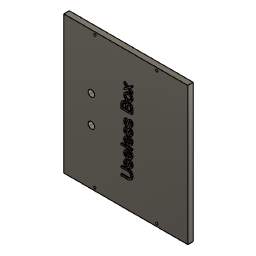
UselessBoxTop v6 (Autodesk Fusion 360 design; units mm, degrees)
Autodesk Fusion 360 part; units mm, degrees
note: some values were not read from the file. Set by a fixed rule: which sketch regions a step uses.
sketch "Sketch1" plane through (0, 0, 0) normal (0, 0, 1) x (1, 0, 0)
  line L0 (0, 0) -> (114.3, 0)
  line L1 (114.3, 0) -> (114.3, 127)
  line L2 (114.3, 127) -> (0, 127)
  line L3 (0, 127) -> (0, 0)
  dimension "d1" = 114.3
  dimension "d2" = 127
  constraint horizontal L0
  constraint vertical L1
  constraint horizontal L2
  constraint vertical L3
  constraint coincident L0.start L3.end
  measures "d1" distance of L0.start L0.end
  measures "d2" distance of L0.start L2.end
extrude "Extrude1" add sketch "Sketch1" along normal blind 5
sketch "Sketch2" plane through (0, 0, 5) normal (0, 0, 1) x (1, 0, 0)
  line L0 (0, 127) -> (0, 0)
  line L1 (0, 0) -> (114.3, 0)
  line L2 (114.3, 0) -> (114.3, 127)
  line L3 (114.3, 127) -> (0, 127)
  line L4 (0, 0) -> (114.3, 0)
  line L5 (114.3, 0) -> (114.3, 2.5)
  line L6 (114.3, 2.5) -> (0, 2.5)
  line L7 (0, 2.5) -> (0, 0)
  line L8 (0, 127) -> (114.3, 127)
  line L9 (114.3, 127) -> (114.3, 124.5)
  line L10 (114.3, 124.5) -> (0, 124.5)
  line L11 (0, 124.5) -> (0, 127)
  line L12 (0, 2.5) -> (28.575, 2.5)
  line L13 (28.575, 2.5) -> (28.575, 0)
  line L14 (28.575, 0) -> (0, 0)
  line L15 (0, 0) -> (0, 2.5)
  line L16 (114.3, 2.5) -> (85.725, 2.5)
  line L17 (85.725, 2.5) -> (85.725, 0)
  line L18 (85.725, 0) -> (114.3, 0)
  line L19 (114.3, 0) -> (114.3, 2.5)
  line L20 (0, 127) -> (28.575, 127)
  line L21 (28.575, 127) -> (28.575, 124.5)
  line L22 (28.575, 124.5) -> (0, 124.5)
  line L23 (0, 124.5) -> (0, 127)
  line L24 (114.3, 124.5) -> (85.725, 124.5)
  line L25 (85.725, 124.5) -> (85.725, 127)
  line L26 (85.725, 127) -> (114.3, 127)
  line L27 (114.3, 127) -> (114.3, 124.5)
  circle A0 centre (28.575, 124.5) radius 1.05
  circle A1 centre (85.725, 124.5) radius 1.05
  circle A2 centre (85.725, 2.5) radius 1.05
  circle A3 centre (28.575, 2.5) radius 1.05
  dimension "d5" = 114.3
  dimension "d6" = 2.5
  dimension "d7" = 114.3
  dimension "d8" = 2.5
  dimension "d9" = 28.575
  dimension "d10" = 28.575
  dimension "d11" = 28.575
  dimension "d12" = 28.575
  dimension "d13" = 2.1
  dimension "d14" = 2.1
  dimension "d15" = 2.1
  dimension "d16" = 2.1
  constraint horizontal L4
  constraint vertical L5
  constraint horizontal L6
  constraint vertical L7
  constraint coincident L0.end L1.start
  constraint horizontal L8
  constraint vertical L9
  constraint horizontal L10
  constraint vertical L11
  constraint coincident L0.start L3.end
  constraint horizontal L12
  constraint vertical L13
  constraint horizontal L14
  constraint vertical L15
  constraint horizontal L16
  constraint vertical L17
  constraint horizontal L18
  constraint vertical L19
  constraint horizontal L20
  constraint vertical L21
  constraint horizontal L22
  constraint vertical L23
  constraint horizontal L24
  constraint vertical L25
  constraint horizontal L26
  constraint vertical L27
  constraint coincident L21.end L22.start
  constraint coincident L24.end L25.start
  constraint coincident L16.end L17.start
  constraint coincident L12.end L13.start
  measures "d5" distance of L0.end L1.end
  measures "d6" distance of L0.end L6.end
  measures "d7" distance of L0.start L2.end
  measures "d8" distance of L0.start L10.end
  measures "d9" distance of L6.end L12.end
  measures "d10" distance of L5.end L16.end
  measures "d11" distance of L0.start L20.end
  measures "d12" distance of L9.end L24.end
  measures "d13" diameter of A0
  measures "d14" diameter of A1
  measures "d15" diameter of A2
  measures "d16" diameter of A3
extrude "Extrude2" cut sketch "Sketch2" against normal blind 5 contours L10 L21 L22 A0 | L10 L22 A0 | L10 L21 A0 | L6 L12 A3 | L6 L12 L13 A3 | L10 L24 L25 A1 | L10 L25 A1 | L6 L13 A3 | L10 L24 A1 | L6 L16 A2 | L6 L17 A2 | L6 L16 L17 A2
sketch "Sketch3" plane through (0, 0, 5) normal (0, 0, 1) x (1, 0, 0)
  circle A0 centre (85.725, 124.5) radius 1.05
  circle A1 centre (85.725, 2.5) radius 1.05
  circle A2 centre (28.575, 124.5) radius 1.05
  circle A3 centre (28.575, 2.5) radius 1.05
  line L0 (0, 127) -> (0, 0)
  line L1 (0, 0) -> (114.3, 0)
  line L2 (114.3, 0) -> (114.3, 127)
  line L3 (114.3, 127) -> (0, 127)
  line L4 (0, 127) -> (25.4, 127)
  line L5 (25.4, 127) -> (25.4, 0)
  line L6 (25.4, 0) -> (0, 0)
  line L7 (0, 0) -> (0, 127)
  line L8 (0, 127) -> (25.4, 127)
  line L9 (25.4, 127) -> (25.4, 76.2)
  line L10 (25.4, 76.2) -> (0, 76.2)
  line L11 (0, 76.2) -> (0, 127)
  line L12 (0, 0) -> (25.4, 0)
  line L13 (25.4, 0) -> (25.4, 50.8)
  line L14 (25.4, 50.8) -> (0, 50.8)
  line L15 (0, 50.8) -> (0, 0)
  circle A4 centre (25.4, 50.8) radius 3
  circle A5 centre (25.4, 76.2) radius 3
  dimension "d19" = 25.4
  dimension "d20" = 50.8
  dimension "d21" = 50.8
  dimension "d22" = 6
  dimension "d23" = 6
  constraint horizontal L4
  constraint vertical L5
  constraint horizontal L6
  constraint vertical L7
  constraint coincident L1 L5.end
  constraint coincident L0.start L3.end
  constraint horizontal L8
  constraint vertical L9
  constraint horizontal L10
  constraint vertical L11
  constraint horizontal L12
  constraint vertical L13
  constraint horizontal L14
  constraint vertical L15
  constraint coincident L13.end L14.start
  constraint coincident L9.end L10.start
  measures "d19" distance of L0.start L4.end
  measures "d20" distance of L0.start L10.end
  measures "d21" distance of L0.end L14.end
  measures "d22" diameter of A4
  measures "d23" diameter of A5
extrude "Extrude3" cut sketch "Sketch3" against normal blind 5 contours L5 L9 L10 A5 | L5 L10 A5 | L5 L9 A5 | L5 L14 A4 | L5 L13 L14 A4 | L5 L13 A4
sketch "Sketch4" plane through (0, 0, 5) normal (0, 0, 1) x (1, 0, 0)
  circle A0 centre (25.4, 76.2) radius 3
  circle A1 centre (25.4, 50.8) radius 3
  circle A2 centre (85.725, 124.5) radius 1.05
  circle A3 centre (85.725, 2.5) radius 1.05
  circle A4 centre (28.575, 124.5) radius 1.05
  circle A5 centre (28.575, 2.5) radius 1.05
  line L0 (0, 127) -> (0, 0)
  line L1 (0, 0) -> (114.3, 0)
  line L2 (114.3, 0) -> (114.3, 127)
  line L3 (114.3, 127) -> (0, 127)
  line L4 (82.2036, 0) -> (82.2036, 127) construction
  line L5 (82.2036, 127) -> (35, 127) construction
  line L6 (35, 127) -> (35, 0) construction
  line L7 (35, 0) -> (82.2036, 0) construction
  dimension "d26" = 10
  text T0 "Useless Box" font "Arial" height 10 align centre middle in box 127 x 47.2036 at (82.2036, 0) x (0, 1) y (-1, 0) spacing 1
  constraint coincident L3
  constraint coincident L1
extrude "Extrude4" add sketch "Sketch4" along normal blind 1 text T0
